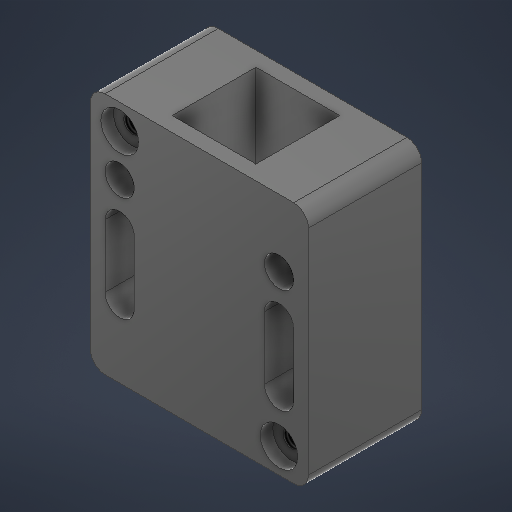
# Autodesk Inventor part: SupportTendeur
Saved by Autodesk Inventor 2026.2 (Build 302298010, 298A)
## iProperties
Created: 2026-04-13
Part Number: SupportTendeur
Material: Générique
Document SubType Name: Modeling
Designer: romai
Density: 1 g/cm^3
Appearance: Par défaut
Author: romai
Autodesk Inventor part; units mm, degrees
ref_plane "YZ Plane" through (0, 0, 0) normal (1, 0, 0) x (0, 1, 0)
ref_plane "XZ Plane" through (0, 0, 0) normal (0, 1, 0) x (-1, 0, 0)
ref_plane "XY Plane" through (0, 0, 0) normal (0, 0, 1) x (1, 0, 0)
sketch "Esquisse1" plane through (0, 0, 0) normal (0, 0, 1) x (1, 0, 0)
  line L0 (22.5, 29) -> (-22.5, 29)
  line L1 (-26, 25.5) -> (-26, -25.5)
  line L2 (-22.5, -29) -> (22.5, -29)
  line L3 (26, -25.5) -> (26, 25.5)
  line L4 (26, 29) -> (-26, -29) construction
  line L5 (-26, 29) -> (26, -29) construction
  line L6 (-19, 6.5) -> (-19, 6.5)
  line L7 (-15.5, 3) -> (-15.5, -12)
  line L8 (-19, -15.5) -> (-19, -15.5)
  line L9 (-22.5, -12) -> (-22.5, 3)
  line L10 (-22.5, 6.5) -> (-15.5, -15.5) construction
  line L11 (-15.5, 6.5) -> (-22.5, -15.5) construction
  circle A0 centre (-19, 13) radius 3.5
  arc A1 (-22.5, -12) -> (-19, -15.5) centre (-19, -12) ccw
  arc A2 (-19, -15.5) -> (-15.5, -12) centre (-19, -12) ccw
  arc A3 (-19, 6.5) -> (-22.5, 3) centre (-19, 3) ccw
  arc A4 (-15.5, 3) -> (-19, 6.5) centre (-19, 3) ccw
  line L12 (0, 45.9017) -> (0, -37.4412)
  line L13 (15.5, 3) -> (15.5, -12)
  line L14 (22.5, -12) -> (22.5, 3)
  circle A5 centre (19, 13) radius 3.5
  arc A6 (19, -15.5) -> (22.5, -12) centre (19, -12) ccw
  arc A7 (15.5, -12) -> (19, -15.5) centre (19, -12) ccw
  arc A8 (22.5, 3) -> (19, 6.5) centre (19, 3) ccw
  arc A9 (19, 6.5) -> (15.5, 3) centre (19, 3) ccw
  arc A10 (-26, -25.5) -> (-22.5, -29) centre (-22.5, -25.5) ccw
  arc A11 (-22.5, 29) -> (-26, 25.5) centre (-22.5, 25.5) ccw
  arc A12 (26, 25.5) -> (22.5, 29) centre (22.5, 25.5) ccw
  arc A13 (22.5, -29) -> (26, -25.5) centre (22.5, -25.5) ccw
  point P0 (0, 0)
  point P1 (-19, -4.5)
  point P2 (19, -15.5)
  point P3 (19, 6.5)
  point P4 (-19, 6.5)
  point P5 (-19, -15.5)
  dimension "d0" = 52
  dimension "d1" = 58
  dimension "d2" = 7
  dimension "d5" = 3.5
  dimension "d6" = 7
  dimension "d7" = 42
  dimension "d8" = 3.5
  dimension "d9" = 15
  dimension "d10" = 17
  dimension "d12" = 0
  dimension "d13" = 3.5
  constraints: 30 end point, 24 point on circle, 16 point on line, 16 tangent, 14 centre point, 13 symmetric about line, 6 equal radius, 4 midpoint, 4 parallel, 2 horizontal, 2 perpendicular, 1 vertical, 5 other
  measures "d0" distance of L4.start L5.start
  measures "d1" distance of L5.start L4.end
  measures "d2" distance of L10.end L11.end
  measures "d5" distance between parallel lines of L1 L9
  measures "d6" diameter of A0
  measures "d7" distance from line of A0.centre L2
  measures "d8" radius of A1
  measures "d9" distance of A2.centre A4.centre
  measures "d10" distance from line of L2 A1.centre
  measures "d12" horizontal distance of A3.centre A0.centre
  measures "d13" radius of A10
extrude "Extrusion1" add sketch "Esquisse1" against normal blind 27
sketch "Esquisse2" plane through (0, 0, 0) normal (0, 0, 1) x (1, 0, 0)
  line L0 (-22.5, -29) -> (22.5, -29) projected
  circle A0 centre (19, 13) radius 3.5 projected
  line L1 (19, 13) -> (19, -23)
  circle A1 centre (-19, 13) radius 3.5 projected
  line L2 (-19, 13) -> (-19, 23)
  line L3 (22.5, 29) -> (-22.5, 29) projected
  point P0 (0, 0)
  dimension "d23" = 6
  dimension "d25" = 6
  constraints: 4 end point, 2 coincident, 2 vertical
  measures "d23" distance from line of L0 L1.end
  measures "d25" distance from line of L3 L2.end
hole "Perçage1" at (19, -23, 0) at (-19, 23, 0) direction (0, 0, -1) diameter 4.134 depth 14.2 counterbore diameter 9 counterbore depth 3 thread size "M5x0.8" class "6H" standard "ANSI Metric M Profile"
sketch "Esquisse3" plane through (-22.5, 29, 0) normal (0, 1, 0) x (1, 0, 0)
  line L0 (45, 0) -> (0, 0) projected
  line L1 (45, 0) -> (45, 27) projected
  line L2 (0, 27) -> (45, 27) projected
  line L3 (0, 0) -> (0, 27) projected
  line L4 (32.5, 3.5) -> (12.5, 3.5)
  line L5 (12.5, 3.5) -> (12.5, 23.5)
  line L6 (12.5, 23.5) -> (32.5, 23.5)
  line L7 (32.5, 23.5) -> (32.5, 3.5)
  line L8 (32.5, 3.5) -> (12.5, 23.5) construction
  line L9 (12.5, 3.5) -> (32.5, 23.5) construction
  point P0 (22.5, 0)
  point P1 (22.5, 13.5)
  dimension "d26" = 20
  dimension "d27" = 20
  constraints: 12 end point, 2 midpoint, 2 parallel, 1 horizontal, 1 perpendicular
  measures "d26" distance of L5.end L6.end
  measures "d27" distance of L4.end L5.end
extrude "Extrusion2" cut sketch "Esquisse3" against normal blind 50 contours L4 L5 L6 L7
